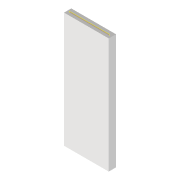
# Autodesk Inventor part: 40_microfluidic_chip_lightsheet_layer1_negative_mould_upper_v0
Saved by Autodesk Inventor 2022 (Build 260153000, 153)
## iProperties
Created: 2021-12-21
Part Number: 40_microfluidic_chip_lightsheet_layer1_negative_mould_upper_v0
Material: Generisch
Document SubType Name: Modeling
Designer: diederichbenedict
Density: 1 g/cm^3
Appearance: Vorgabe
Author: diederichbenedict
Autodesk Inventor part; units mm, degrees
ref_plane "YZ Plane" through (0, 0, 0) normal (1, 0, 0) x (0, 1, 0)
ref_plane "XZ Plane" through (0, 0, 0) normal (0, 1, 0) x (-1, 0, 0)
ref_plane "Arbeitsebene1" through (0, 0, 0) normal (0, 0, 1) x (1, 0, 0)
sketch "Skizze1" plane through (0, 0, 0) normal (0, 0, 1) x (1, 0, 0)
  line L0 (12.5, -37) -> (-12.5, -37) projected
  line L1 (12.5, 37) -> (12.5, -37) projected
  line L2 (-12.5, 37) -> (12.5, 37) projected
  line L3 (-12.5, -37) -> (-12.5, 37) projected
  circle A0 centre (-8.5, -30) radius 1.4 projected
  circle A1 centre (8.5, -30) radius 1.4 projected
  circle A2 centre (8.5, 30) radius 1.4 projected
  circle A3 centre (-8.5, 30) radius 1.4 projected
  line L4 (-0.75, 23.146) -> (-0.75, -23.146) projected
  arc A4 (0.75, 23.146) -> (-0.75, 23.146) centre (0, 25) ccw projected
  line L5 (0.75, -23.146) -> (0.75, 23.146) projected
  arc A5 (-0.75, -23.146) -> (0.75, -23.146) centre (0, -25) ccw projected
  line L6 (15.5, -40) -> (-15.5, -40)
  line L7 (-15.5, -40) -> (-15.5, 40)
  line L8 (-15.5, 40) -> (15.5, 40)
  line L9 (15.5, 40) -> (15.5, -40)
  point P0 (0, 0)
  dimension "d0" = 3
  constraints: 8 end point, 3 other
  measures "d0" distance between parallel lines of L1 L9
extrude "Extrusion1" add sketch "Skizze1" along normal blind 2 contours L0 L3 L2 L1 | A0 | A1 | A2 | A3 | A4 L5 A5 L4 | L6 L7 L8 L9
ref_plane "Arbeitsebene2" through (-2, 9.25, -0.4) normal (0, 0, 1) x (1, 0, 0)
sketch "Skizze2" plane through (0, 0, 0) normal (0, 0, -1) x (-1, 0, 0)
  circle A0 centre (0, -25) radius 2.5 construction
  circle A1 centre (0, 25) radius 2.5 construction
  line L0 (12.5, -37) -> (12.5, 37)
  line L1 (12.5, 37) -> (-12.5, 37)
  line L2 (-12.5, 37) -> (-12.5, -37)
  line L3 (-12.5, -37) -> (12.5, -37)
  circle A2 centre (8.5, -30) radius 1.4
  circle A3 centre (-8.5, -30) radius 1.4
  circle A4 centre (-8.5, 30) radius 1.4
  circle A5 centre (8.5, 30) radius 1.4
  line L4 (0.75, -7.25) -> (0.75, -23.146) construction
  line L5 (-0.75, 7.25) -> (-0.75, 23.146) construction
  line L6 (0.75, -7.25) -> (0.75, -23.146) construction
  line L7 (-0.75, 7.25) -> (-0.75, 23.146) construction
  circle A6 centre (0, -25) radius 2.5 construction
  circle A7 centre (0, 25) radius 2.5 construction
  circle A8 centre (0, 25) radius 32.2587 construction
  circle A9 centre (0, -25) radius 2 construction
  circle A10 centre (0, 25) radius 1.5
  circle A11 centre (0, -25) radius 1.5
  line L8 (0.75, 23.701) -> (-0.75, 23.701)
  line L9 (-0.75, 23.701) -> (-0.75, -23.701)
  line L10 (-0.75, -23.701) -> (0.75, -23.701)
  line L11 (0.75, -23.701) -> (0.75, 23.701)
  line L12 (-9.25, 9.25) -> (9.25, 9.25)
  line L13 (9.25, 9.25) -> (9.25, -9.25)
  line L14 (9.25, -9.25) -> (-9.25, -9.25)
  line L15 (-9.25, -9.25) -> (-9.25, 9.25)
  point P0 (0, 0)
  point P1 (-0.75, 22.6152)
  point P2 (-0.75, -22.6152)
  point P3 (0.75, -22.6152)
  point P4 (0.75, 22.6152)
  point P5 (-0.75, -23.146)
extrude "Extrusion2" add sketch "Skizze2" along normal blind 0.5 contours A2 | A3 | A4 | A5 | A10 L8 | L8 A10 | A10 L11 L12 L9 | L12 L11 L14 L9 | L14 L11 A11 L9 | L10 A11 picked at (0.3855, -25.1784)
sketch "Skizze4" plane through (0, 0, 0) normal (0, 0, -1) x (-1, 0, 0)
  circle A0 centre (8.5, -30) radius 1.4 projected
  circle A1 centre (-8.5, 30) radius 1.4 projected
  arc A2 (0.75, 23.701) -> (-0.75, 23.701) centre (0, 25) ccw projected
  line L0 (0.75, 23.701) -> (0.75, -23.701) projected
  arc A3 (-0.75, -23.701) -> (0.75, -23.701) centre (0, -25) ccw projected
  line L1 (-0.75, -23.701) -> (-0.75, 23.701) projected
  circle A4 centre (-8.5, -30) radius 1.4 projected
  circle A5 centre (8.5, 30) radius 1.4 projected
  line L2 (-15.5, 40) -> (15.5, 40) projected
  line L3 (-15.5, -40) -> (-15.5, 40) projected
  line L4 (15.5, -40) -> (-15.5, -40) projected
  line L5 (15.5, 40) -> (15.5, -40) projected
  line L6 (12.65, 37.15) -> (-12.65, 37.15)
  line L7 (-12.65, 37.15) -> (-12.65, -37.15)
  line L8 (-12.65, -37.15) -> (12.65, -37.15)
  line L9 (12.65, -37.15) -> (12.65, 37.15)
  point P0 (0, 0)
  dimension "d11" = 2.85
  constraints: 8 end point, 3 other
  measures "d11" distance between parallel lines of L2 L6
extrude "Extrusion4" add sketch "Skizze4" along normal blind 3 contours L2 L5 L4 L3
